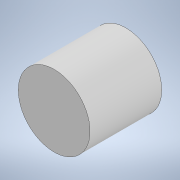
# Autodesk Inventor part: Layout
Saved by Autodesk Inventor 2022 (Build 260153070, 153G)
## iProperties
Created: 2021-11-12
Part Number: Layout
Material: Generic
Document SubType Name: Modeling
Designer: elmar
Density: 1 g/cm^3
Appearance: Default
Author: elmar
Autodesk Inventor part; units mm, degrees
ref_plane "YZ Plane" through (0, 0, 0) normal (1, 0, 0) x (0, 1, 0)
ref_plane "XZ Plane" through (0, 0, 0) normal (0, 1, 0) x (-1, 0, 0)
ref_plane "XY Plane" through (0, 0, 0) normal (0, 0, 1) x (1, 0, 0)
sketch "Sketch1" plane through (0, 0, 0) normal (0, 0, 1) x (1, 0, 0)
  circle A0 centre (0, 0) radius 203
  line L0 (-129, -156.7418) -> (-129, -267)
  line L1 (-129, -267) -> (129, -267)
  line L2 (129, -267) -> (129, -156.7418)
  circle A1 centre (0, 0) radius 37
  dimension "d0" = 406
  dimension "d1" = 267
  dimension "d2" = 74
  dimension "d3" = 258
  constraints: 6 end point, 2 centre point, 2 coincident, 2 perpendicular, 2 point on circle, 1 parallel, 1 vertical
  measures "d0" diameter of A0
  measures "d1" distance from line of L1 point (0, 0)
  measures "d2" diameter of A1
  measures "d3" distance of L0.end L1.end
extrude "Extrusion1" add sketch "Sketch1" along normal blind 74 contours A1
body "Solid1"
